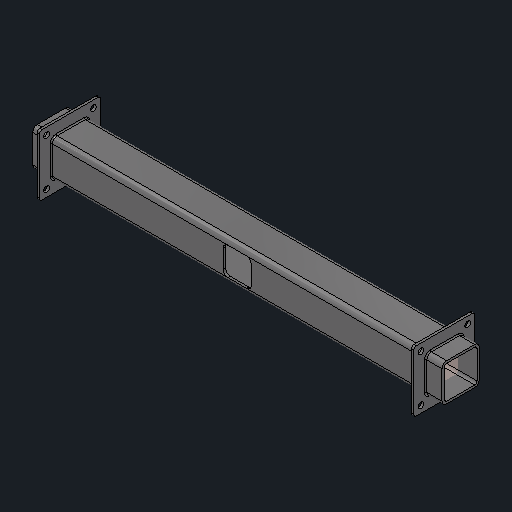
# Autodesk Inventor part: Model-3_Base Tube-1
Saved by Autodesk Inventor 2025.1 (Build 291241000, 241)
## iProperties
RuleStatus: InUse
Created: 2026-02-13
Part Number: Model-3_Base Tube-1
User Status: Released
Material: SS304
Description: Model-1 Base Tube-1
Document SubType Name: Modeling
Designer: Desktop -24
Density: 7.99949 g/cm^3
Appearance: Semi-Polished(1)
Mass: 20583.6 g
Surface Area: 8150.6 cm^2
Volume: 2573.11 cm^3
AfterDocNew0: Mat. Selection
encoded128: ÌStandard Î
encoded39: *STANDARD*
Family: SS304
Author: Desktop -24
Revision Number: 0
Autodesk Inventor part; units mm, degrees
ref_plane "YZ Plane" through (0, 0, 0) normal (1, 0, 0) x (0, 1, 0)
ref_plane "XZ Plane" through (0, 0, 0) normal (0, 1, 0) x (-1, 0, 0)
ref_plane "XY Plane" through (0, 0, 0) normal (0, 0, 1) x (1, 0, 0)
sketch "Sketch5" plane through (0, 0, 0) normal (1, 0, 0) x (0, 1, 0)
  line L0 (-38.1, 50.8) -> (38.1, 50.8)
  line L1 (50.8, 38.1) -> (50.8, -38.1)
  line L2 (38.1, -50.8) -> (-38.1, -50.8)
  line L3 (-50.8, -38.1) -> (-50.8, 38.1)
  line L4 (-50.8, 50.8) -> (50.8, -50.8) construction
  line L5 (50.8, 50.8) -> (-50.8, -50.8) construction
  arc A0 (50.8, 38.1) -> (38.1, 50.8) centre (38.1, 38.1) ccw
  arc A1 (38.1, -50.8) -> (50.8, -38.1) centre (38.1, -38.1) ccw
  arc A2 (-50.8, -38.1) -> (-38.1, -50.8) centre (-38.1, -38.1) ccw
  arc A3 (-38.1, 50.8) -> (-50.8, 38.1) centre (-38.1, 38.1) ccw
  line L6 (44.45, -38.1) -> (44.45, 38.1)
  arc A4 (44.45, 38.1) -> (38.1, 44.45) centre (38.1, 38.1) ccw
  line L7 (38.1, 44.45) -> (-38.1, 44.45)
  arc A5 (-38.1, 44.45) -> (-44.45, 38.1) centre (-38.1, 38.1) ccw
  line L8 (-44.45, 38.1) -> (-44.45, -38.1)
  arc A6 (-44.45, -38.1) -> (-38.1, -44.45) centre (-38.1, -38.1) ccw
  line L9 (-38.1, -44.45) -> (38.1, -44.45)
  arc A7 (38.1, -44.45) -> (44.45, -38.1) centre (38.1, -38.1) ccw
  point P0 (0, 0)
  dimension "d6" = 101.6
  dimension "d7" = 101.6
  dimension "d8" = 12.7
  dimension "d9" = 6.35
  constraints: 20 end point, 16 point on circle, 8 centre point, 8 point on line, 8 tangent, 4 parallel, 3 equal radius, 2 midpoint, 2 perpendicular, 1 horizontal, 7 other
  measures "d6" distance of L5.start L4.end
  measures "d7" distance of L4.end L5.end
  measures "d8" radius of A0
  measures "d9" distance between parallel lines of L1 L6
extrude "Extrusion4" add sketch "Sketch5" along normal mid plane 1111.25
sketch "Sketch6" plane through (-555.625, -38.1, 50.8) normal (0, 0, 1) x (1, 0, 0)
  line L0 (530.225, 0) -> (581.025, 0)
  line L1 (593.725, 12.7) -> (593.725, 63.5)
  line L2 (581.025, 76.2) -> (530.225, 76.2)
  line L3 (517.525, 63.5) -> (517.525, 12.7)
  line L4 (517.525, 0) -> (593.725, 76.2) construction
  line L5 (593.725, 0) -> (517.525, 76.2) construction
  arc A0 (530.225, 76.2) -> (517.525, 63.5) centre (530.225, 63.5) ccw
  arc A1 (593.725, 63.5) -> (581.025, 76.2) centre (581.025, 63.5) ccw
  arc A2 (517.525, 12.7) -> (530.225, 0) centre (530.225, 12.7) ccw
  arc A3 (581.025, 0) -> (593.725, 12.7) centre (581.025, 12.7) ccw
  point P0 (555.625, 38.1)
  dimension "d12" = 76.2
  dimension "d13" = 76.2
  dimension "d14" = 12.7
  constraints: 12 end point, 8 point on circle, 8 point on line, 8 tangent, 4 centre point, 3 equal radius, 2 midpoint, 2 parallel, 1 horizontal, 1 perpendicular
  measures "d12" distance of L4.end L5.end
  measures "d13" distance of L5.start L4.end
  measures "d14" radius of A0
extrude "Extrusion5" cut sketch "Sketch6" against normal blind 177.8
ref_plane "Work Plane1" through (504.825, 0, 0) normal (1, 0, 0) x (0, 0, -1)
sketch "Sketch7" plane through (504.825, 0, 0) normal (1, 0, 0) x (0, 0, -1)
  line L0 (-76.2, -82.55) -> (76.2, -82.55)
  line L1 (82.55, -76.2) -> (82.55, 76.2)
  line L2 (76.2, 82.55) -> (-76.2, 82.55)
  line L3 (-82.55, 76.2) -> (-82.55, -76.2)
  line L4 (-82.55, -82.55) -> (82.55, 82.55) construction
  line L5 (82.55, -82.55) -> (-82.55, 82.55) construction
  line L6 (38.1, 50.8) -> (-38.1, 50.8) projected
  line L7 (50.8, -38.1) -> (50.8, 38.1) projected
  arc A0 (-76.2, 82.55) -> (-82.55, 76.2) centre (-76.2, 76.2) ccw
  arc A1 (82.55, 76.2) -> (76.2, 82.55) centre (76.2, 76.2) ccw
  arc A2 (76.2, -82.55) -> (82.55, -76.2) centre (76.2, -76.2) ccw
  arc A3 (-82.55, -76.2) -> (-76.2, -82.55) centre (-76.2, -76.2) ccw
  arc A4 (-38.1, 50.8) -> (-50.8, 38.1) centre (-38.1, 38.1) ccw projected
  arc A5 (50.8, 38.1) -> (38.1, 50.8) centre (38.1, 38.1) ccw projected
  arc A6 (38.1, -50.8) -> (50.8, -38.1) centre (38.1, -38.1) ccw projected
  line L8 (-38.1, -50.8) -> (38.1, -50.8) projected
  arc A7 (-50.8, -38.1) -> (-38.1, -50.8) centre (-38.1, -38.1) ccw projected
  line L9 (-50.8, 38.1) -> (-50.8, -38.1) projected
  point P0 (0, 0)
  dimension "d17" = 31.75
  dimension "d18" = 31.75
  dimension "d19" = 6.35
  constraints: 12 end point, 8 point on circle, 8 point on line, 8 tangent, 4 centre point, 3 equal radius, 2 midpoint, 2 parallel, 1 horizontal, 1 perpendicular
  measures "d17" distance between parallel lines of L6 L2
  measures "d18" distance between parallel lines of L1 L7
  measures "d19" radius of A0
extrude "Extrusion6" add sketch "Sketch7" along normal blind 6.35
fillet "Fillet1" radius 3.175 16 edges at (504.825, 47.0803, -47.0803) (504.825, 0, -50.8) (504.825, -47.0803, -47.0803) (504.825, -50.8, 0) (504.825, -47.0803, 47.0803) (504.825, 0, 50.8) (504.825, 47.0803, 47.0803) (504.825, 50.8, 0) (511.175, 47.0803, 47.0803) (511.175, 0, 50.8) (511.175, -47.0803, 47.0803) (511.175, -50.8, 0) (511.175, -47.0803, -47.0803) (511.175, 0, -50.8) (511.175, 47.0803, -47.0803) (511.175, 50.8, 0)
sketch "Sketch8" plane through (511.175, 0, 0) normal (1, 0, 0) x (0, 0, -1)
  line L0 (-63.5, -63.5) -> (63.5, -63.5) construction
  line L1 (63.5, -63.5) -> (63.5, 63.5) construction
  line L2 (63.5, 63.5) -> (-63.5, 63.5) construction
  line L3 (-63.5, 63.5) -> (-63.5, -63.5) construction
  line L4 (-63.5, -63.5) -> (63.5, 63.5) construction
  line L5 (63.5, -63.5) -> (-63.5, 63.5) construction
  line L6 (76.2, 82.55) -> (-76.2, 82.55) projected
  line L7 (82.55, -76.2) -> (82.55, 76.2) construction
  circle A0 centre (-63.5, 63.5) radius 7.9375
  circle A1 centre (63.5, 63.5) radius 7.9375
  circle A2 centre (63.5, -63.5) radius 7.9375
  circle A3 centre (-63.5, -63.5) radius 7.9375
  point P0 (0, 0)
  dimension "d23" = 19.05
  dimension "d24" = 19.05
  dimension "d25" = 15.875
  constraints: 12 end point, 4 centre point, 4 coincident, 3 equal radius, 2 midpoint, 2 parallel, 1 horizontal, 1 perpendicular
  measures "d23" distance between parallel lines of L6 L2
  measures "d24" distance between parallel lines of L7 L1
  measures "d25" diameter of A0
extrude "Extrusion7" cut sketch "Sketch8" against normal blind 6.35
mirror "Mirror2" about plane through (0, 0, 0) normal (1, 0, 0) of "Extrusion7", "Fillet1", "Extrusion6"
equation "\"d18\" = d17"
equation "\"d24\" = d23"
body "Solid4"
